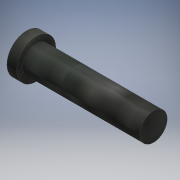
# Autodesk Inventor part: bolt_M2L6
Saved by Autodesk Inventor 2017.3 (Build 213256000, 256)
## iProperties
Part Number: bolt_M2L6
Material: 鋼
Document SubType Name: Modeling
Designer: sktom
Density: 7.85 g/cm^3
Appearance: プレート
Author: sktom
Autodesk Inventor part; units mm, degrees
ref_plane "YZ Plane" through (0, 0, 0) normal (1, 0, 0) x (0, 1, 0)
ref_plane "XZ Plane" through (0, 0, 0) normal (0, 1, 0) x (-1, 0, 0)
ref_plane "XY Plane" through (0, 0, 0) normal (0, 0, 1) x (1, 0, 0)
sketch "スケッチ1" plane through (0, 0, 0) normal (0, 0, 1) x (1, 0, 0)
  line L0 (0, 0) -> (6.5, 0)
  line L1 (6.5, 0) -> (6.5, 0.7)
  line L2 (6.5, 0.7) -> (0.5, 0.7)
  line L3 (0.5, 0.7) -> (0.5, 1)
  line L4 (0.5, 1) -> (0, 1)
  line L5 (0, 1) -> (0, 0)
  dimension "d0" = 0.5
  dimension "d1" = 1
  dimension "d2" = 0.7
  dimension "d3" = 6
  constraints: 12 end point, 5 perpendicular, 1 horizontal
  measures "d0" distance of L3.end L4.end
  measures "d1" distance between parallel lines of L0 L4
  measures "d2" distance of L0.end L1.end
  measures "d3" distance of L1.end L2.end
revolve "回転1" add sketch "スケッチ1" angle 360 about axis through (0, 0, 0) along (1, 0, 0)
